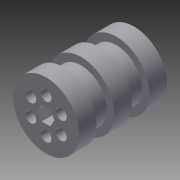
# Autodesk Inventor part: WheelHub
Saved by Autodesk Inventor 2012 (Build 160160000, 160)
## iProperties
Created: 2012-02-07
Part Number: WheelHub
Material: Aluminum-6061
Document SubType Name: Modeling
Designer: admin
Mass: 41.11 g
Surface Area: 93.8702 cm^2
Volume: 15.1698 cm^3
Density: 2.71 g/cm^3
Author: admin
Autodesk Inventor part; units mm, degrees
ref_plane "YZ Plane" through (0, 0, 0) normal (1, 0, 0) x (0, 1, 0)
ref_plane "XZ Plane" through (0, 0, 0) normal (0, 1, 0) x (-1, 0, 0)
sketch "Sketch1" plane through (0, 0, 0) normal (0, 0, 1) x (1, 0, 0)
  line L0 (-1.8331, 3.175) -> (1.8331, 3.175)
  line L1 (1.8331, 3.175) -> (3.6662, 0)
  line L2 (3.6662, 0) -> (1.8331, -3.175)
  line L3 (1.8331, -3.175) -> (-1.8331, -3.175)
  line L4 (-1.8331, -3.175) -> (-3.6662, 0)
  line L5 (-3.6662, 0) -> (-1.8331, 3.175)
  circle A0 centre (0, 0) radius 14.2875
  dimension "d1" = 6.35
  dimension "d4" = 28.575
  constraints: 12 end point, 2 coincident, 1 centre point, 1 horizontal, 13 other
  measures "d1" distance between parallel lines of L3 L0
  measures "d4" diameter of A0
extrude "Extrusion1" add sketch "Sketch1" along normal mid plane 38.1
ref_plane "Work Plane5" through (-2.7496, 1.5875, -11.43) normal (0, 0, 1) x (1, 0, 0)
ref_plane "Work Plane4" through (-2.7496, 1.5875, -3.81) normal (0, 0, 1) x (1, 0, 0)
sketch "Sketch2" plane through (-2.7496, 1.5875, 11.43) normal (0, 0, 1) x (1, 0, 0)
  circle A0 centre (2.7496, -1.5875) radius 11.1125
  circle A1 centre (2.7496, -1.5875) radius 14.2875 projected
  dimension "d9" = 22.225
  constraints: 1 centre point, 1 coincident
  measures "d9" diameter of A0
extrude "Extrusion2" cut sketch "Sketch2" against normal blind 7.62
sketch "Sketch3" plane through (-2.7496, 1.5875, -3.81) normal (0, 0, 1) x (1, 0, 0)
  circle A0 centre (2.7496, -1.5875) radius 14.2875 projected
  circle A1 centre (2.7496, -1.5875) radius 11.1125 projected
  point P0 (2.7351, -1.6125)
sketch "Sketch4" plane through (0, 0, -19.05) normal (0, 0, -1) x (-1, 0, 0)
  circle A0 centre (0, 0) radius 14.2875 projected
  point P0 (0, 7.62)
  point P1 (-6.5991, 3.81)
  point P2 (-6.5991, -3.81)
  point P3 (0, -7.62)
  point P4 (6.5991, -3.81)
  point P5 (6.5991, 3.81)
  dimension "d15" = 7.62
  dimension "d18" = 360
  constraints: 7 other
  measures "d15" distance of A0.centre point (0, 7.62)
hole "Hole1" at (0, 7.62, -19.05) at (6.5991, 3.81, -19.05) at (6.5991, -3.81, -19.05) at (0, -7.62, -19.05) at (-6.5991, -3.81, -19.05) at (-6.5991, 3.81, -19.05) direction (0, 0, 1) diameter 4.7625 end through all
extrude "Extrusion4" cut sketch "Sketch3" against normal blind 7.62
ref_plane "Work Plane1" through (-2.7496, 1.5875, 19.05) normal (0, 0, 1) x (1, 0, 0)
ref_plane "Work Plane2" through (-2.7496, 1.5875, 11.43) normal (0, 0, 1) x (1, 0, 0)
ref_plane "Work Plane3" through (-2.7496, 1.5875, 3.81) normal (0, 0, 1) x (1, 0, 0)
body "Solid1"
